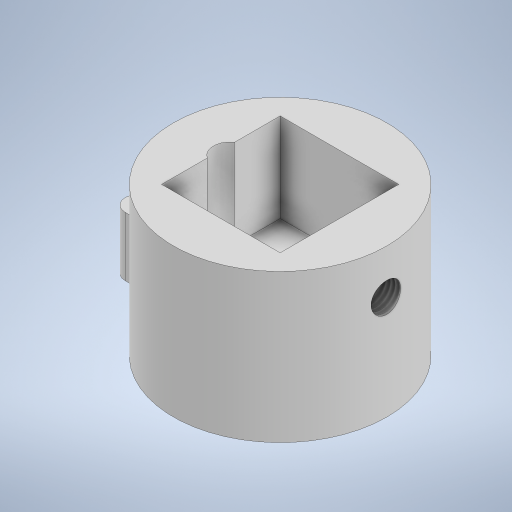
# Autodesk Inventor part: antenna_polarization_rot_conn
Saved by Autodesk Inventor 2024 (Build 280153000, 153)
## iProperties
Created: 2025-12-27
Part Number: antenna_polarization_rot_conn
Material: Generic
Document SubType Name: Modeling
Designer: schar
Density: 1 g/cm^3
Appearance: Default
Author: schar
Autodesk Inventor part; units mm, degrees
note: some values were not read from the file. Chosen so that the rebuilt part matches the saved one: second side of "Extrusion5".
ref_plane "Work Plane1" through (-34, 46.7, -2.9) normal (0, 1, 0) x (1, 0, 0)
sketch "Sketch1" plane through (-34, 46.7, -2.9) normal (0, 1, 0) x (1, 0, 0)
  line L0 (14, 7.1) -> (34, 7.1)
  line L1 (34, 7.1) -> (34, -12.9)
  line L2 (34, -12.9) -> (14, -12.9)
  line L3 (14, -12.9) -> (14, 7.1)
  arc A0 (25.6248, -2.4) -> (22.3752, -2.4) centre (24, -2.9) ccw projected
  line L4 (14, 7.1) -> (34, -12.9) construction
  line L5 (34, 7.1) -> (14, -12.9) construction
  circle A1 centre (24, -2.9) radius 18
  line L6 (6, -6.65) -> (6, 0.85) projected
  arc A2 (4.208, -3.9167) -> (4.9845, -2.5719) centre (4, -2.9) ccw projected
  circle A3 centre (4, -2.9) radius 1
  circle A4 centre (0, -2.9) radius 1.5377
  circle A5 centre (0, -2.9) radius 2.15
  line L7 (0, -0.75) -> (6.126, -0.774)
  line L8 (0, -5.05) -> (6.126, -5.026)
  circle A6 centre (15.4874, -2.9) radius 1.0064
  circle A7 centre (0, -2.9) radius 1
  point P0 (34, -2.9)
  point P1 (6, -5.0265)
  point P2 (6, -2.9)
  point P3 (6, -0.7735)
  dimension "d1" = 20
  dimension "d2" = 20
  dimension "d3" = 2
  dimension "d4" = 4.3
  dimension "d15" = 2
  constraints: 16 end point, 6 centre point, 5 coincident, 4 point on circle, 2 midpoint, 2 parallel, 1 horizontal, 1 perpendicular, 1 tangent
  measures "d1" distance of L1.end L2.end
  measures "d2" distance of L0.end L1.end
  measures "d3" diameter of A3
  measures "d4" diameter of A5
  measures "d15" diameter of A7
extrude "Extrusion1" add sketch "Sketch1" along normal blind 10 contours L0 L1 L2 L3 | A1 | L6 L8 A5 L7 | A4 | A7
sketch "Sketch2" plane through (-10, 56.7, 0) normal (0, 1, 0) x (1, 0, 0)
  line L0 (-10, 10) -> (10, 10)
  line L1 (10, 10) -> (10, -10)
  line L2 (10, -10) -> (-10, -10)
  line L3 (-10, -10) -> (-10, 10)
  circle A0 centre (0, 0) radius 1.25 projected
  line L4 (-10, 10) -> (10, -10) construction
  line L5 (10, 10) -> (-10, -10) construction
  point P0 (10, 0)
  dimension "d7" = 20
  dimension "d8" = 20
  constraints: 12 end point, 2 midpoint, 2 parallel, 1 horizontal, 1 perpendicular
  measures "d7" distance of L1.end L2.end
  measures "d8" distance of L0.end L1.end
extrude "Extrusion2" cut sketch "Sketch2" against normal blind 5
ref_plane "Work Plane6" through (-10, 56.7, 0) normal (0, 1, 0) x (1, 0, 0)
sketch "Sketch3" plane through (-10, 56.7, 0) normal (0, 1, 0) x (1, 0, 0)
  arc A0 (-17.7649, -2.9) -> (-17.7649, 2.9) centre (0, 0) ccw projected
  line L0 (-12.4382, 13.0112) -> (12.4382, 13.0112)
  line L1 (12.4382, 13.0112) -> (12.4382, -13.0112)
  line L2 (12.4382, -13.0112) -> (-12.4382, -13.0112)
  line L3 (-12.4382, -13.0112) -> (-12.4382, 13.0112)
  line L4 (-12.4382, 13.0112) -> (12.4382, -13.0112) construction
  line L5 (12.4382, 13.0112) -> (-12.4382, -13.0112) construction
  line L6 (10, 10) -> (10, -10) projected
  line L7 (-10, 10) -> (10, 10)
  line L8 (10, 10) -> (10, -10)
  line L9 (10, -10) -> (-10, -10)
  line L10 (-10, -10) -> (-10, 10)
  arc A1 (-5.1875, -1.8275) -> (-1.8275, -5.1875) centre (0, 0) ccw projected
  line L11 (-10, 10) -> (10, -10) construction
  line L12 (10, 10) -> (-10, -10) construction
  point P0 (10, 0)
  point P1 (0, 0)
  constraints: 24 end point, 4 midpoint, 4 parallel, 2 horizontal, 2 perpendicular, 1 point on circle
extrude "Extrusion3" add sketch "Sketch3" along normal blind 15 contours L3 L0 L1 L2
ref_plane "Work Plane5" through (-34, 46.7, 0) normal (0, -1, 0) x (1, 0, 0)
sketch "Sketch5" plane through (-34, 46.7, 0) normal (0, -1, 0) x (1, 0, 0)
  circle A0 centre (0, 0) radius 1
  point P0 (34, 0)
  dimension "d16" = 2
  constraints: 1 centre point
  measures "d16" diameter of A0
extrude "Extrusion4" cut sketch "Sketch5" against normal through all
sketch "Sketch6" plane through (-10, 51.7, 0) normal (0, 1, 0) x (1, 0, 0)
  arc A0 (-7.634, 0.5) -> (-7.634, -0.5) centre (-8.5, 0) ccw projected
  circle A1 centre (-8.5, 0) radius 2.75
  point P0 (10, 0)
  dimension "d19" = 5.5
  constraints: 1 centre point, 1 coincident
  measures "d19" diameter of A1
extrude "Extrusion5" cut sketch "Sketch6" along normal blind 20
sketch "Sketch7" plane through (-10, 56.7, 0) normal (0, 1, 0) x (1, 0, 0)
  circle A0 centre (0, 0) radius 1.25
  point P0 (10, 0)
  constraints: 1 centre point
extrude "Extrusion6" cut sketch "Sketch7" against normal up to surface (10 mm away)
ref_plane "Work Plane7" through (-10, 51.7, 0) normal (0, 1, 0) x (1, 0, 0)
sketch "Sketch9" plane through (-10, 51.7, 0) normal (0, 1, 0) x (1, 0, 0)
  line L0 (10, 10) -> (10, -10) projected
  line L1 (-10, 10) -> (10, 10)
  line L2 (10, 10) -> (10, -10)
  line L3 (10, -10) -> (-10, -10)
  line L4 (-10, -10) -> (-10, 10)
  line L5 (-10, 10) -> (10, -10) construction
  line L6 (10, 10) -> (-10, -10) construction
  arc A0 (-7.634, 0.5) -> (-7.634, -0.5) centre (-8.5, 0) ccw projected
  circle A1 centre (-8.5, 0) radius 2.75
  circle A2 centre (0, 0) radius 2.75
  point P0 (10, 0)
  point P1 (-10, 2.3049)
  point P2 (-10, -2.3049)
  dimension "d26" = 5.5
  constraints: 12 end point, 2 centre point, 2 coincident, 2 midpoint, 2 parallel, 1 horizontal, 1 perpendicular
  measures "d26" diameter of A2
extrude "Extrusion7" add sketch "Sketch9" along normal blind 5 contours L0 L3 L4 A1 L1
ref_plane "Work Plane4" through (-34, 56.7, -2.9) normal (0, 1, 0) x (1, 0, 0)
sketch "Sketch10" plane through (-34, 56.7, -2.9) normal (0, 1, 0) x (1, 0, 0)
  arc A0 (21.2958, -3.4) -> (26.7042, -3.4) centre (24, -2.9) ccw projected
  circle A1 centre (24, -2.9) radius 18
  line L0 (36.4382, -15.9112) -> (36.4382, 10.1112) projected
  line L1 (11.5618, 10.1112) -> (36.4382, 10.1112)
  line L2 (36.4382, 10.1112) -> (36.4382, -15.9112)
  line L3 (36.4382, -15.9112) -> (11.5618, -15.9112)
  line L4 (11.5618, -15.9112) -> (11.5618, 10.1112)
  line L5 (11.5618, 10.1112) -> (36.4382, -15.9112) construction
  line L6 (36.4382, 10.1112) -> (11.5618, -15.9112) construction
  point P0 (34, -2.9)
  constraints: 12 end point, 2 midpoint, 2 parallel, 1 centre point, 1 coincident, 1 horizontal, 1 perpendicular
extrude "Extrusion8" add sketch "Sketch10" along normal blind 15 contours A1 L0 | L1 A1 | A1 L3 | L4 A1
ref_plane "Work Plane8" through (0, 71.7, -10) normal (-1, 0, 0) x (0, 0, 1)
sketch "Sketch11" plane through (0, 71.7, -10) normal (-1, 0, 0) x (0, 0, 1)
  line L0 (0, 0) -> (20, 0) projected
  line L1 (10, 0) -> (10, -7.5)
  circle A0 centre (10, -7.5) radius 2.5
  point P0 (10, -71.7)
  dimension "d31" = 7.5
  dimension "d32" = 5
  constraints: 2 end point, 1 centre point, 1 coincident, 1 midpoint, 1 vertical
  measures "d31" distance of L1.start L1.end
  measures "d32" diameter of A0
extrude "Extrusion9" cut sketch "Sketch11" against normal through all
ref_plane "Work Plane2" through (-34, 46.7, 0) normal (0, 1, 0) x (1, 0, 0)
sketch "Sketch12" plane through (-34, 46.7, 0) normal (0, 1, 0) x (1, 0, 0)
  line L0 (6, -2.1265) -> (0, -2.15) projected
  line L1 (6, -2.1265) -> (6.1261, -2.1265)
  arc A0 (6, 0) -> (6.2351, -2.9) centre (24, 0) ccw projected
  line L2 (6, 3.75) -> (6, -3.75) projected
  line L3 (6, 2.1276) -> (6.1261, 2.1276)
  point P0 (34, 0)
  constraints: 4 end point, 1 horizontal, 1 perpendicular, 1 point on circle, 1 point on line
extrude "Extrusion10" add sketch "Sketch12" along normal blind 10
ref_plane "Work Plane3" through (-34, 46.7, 0) normal (0, 1, 0) x (1, 0, 0)
sketch "Sketch13" plane through (-34, 46.7, 0) normal (0, 1, 0) x (1, 0, 0)
  line L0 (0, 2.15) -> (6, 2.1265) projected
  line L1 (6, 2.1265) -> (6.1261, 2.1265)
  arc A0 (6.2351, 2.9) -> (6, 0) centre (24, 0) ccw projected
  line L2 (6.2, -3.55) -> (6.2, 3.55) projected
  line L3 (6, 2.1265) -> (6.2, 2.1265)
  line L4 (6.2, 2.1265) -> (6.2, 0)
  line L5 (6.2, 0) -> (6, 0)
  line L6 (6, 0) -> (6, 2.1265)
  point P0 (34, 0)
  point P1 (6, 0)
  constraints: 10 end point, 2 horizontal, 2 parallel, 1 midpoint, 1 perpendicular, 1 point on circle
extrude "Extrusion11" add sketch "Sketch13" along normal blind 10 contours L1 A0 L6
thread "Thread2" size "M5x0.8" class "6H" standard "ANSI Metric M Profile" length 15
thread "Thread3" size "M2.2x0.45" class "6H" standard "ANSI Metric M Profile" length 15
thread "Thread4" size "M2.5x0.45" class "6H" standard "ANSI Metric M Profile" length 15
body "Solid1"
